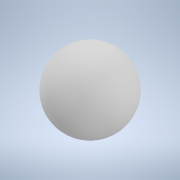
# Autodesk Inventor part: Ball 4mm
Saved by Autodesk Inventor 2021 (Build 250183000, 183)
## iProperties
Created: 2021-08-24
Part Number: Ball 4mm
Material: Genérico
Document SubType Name: Modeling
Designer: Diego.labarca
Density: 1 g/cm^3
Appearance: Valor por defecto
Author: Diego.labarca
Autodesk Inventor part; units mm, degrees
ref_plane "YZ Plane" through (0, 0, 0) normal (1, 0, 0) x (0, 1, 0)
ref_plane "XZ Plane" through (0, 0, 0) normal (0, 1, 0) x (-1, 0, 0)
ref_plane "XY Plane" through (0, 0, 0) normal (0, 0, 1) x (1, 0, 0)
sketch "Boceto1" plane through (0, 0, 0) normal (0, 0, 1) x (1, 0, 0)
  line L0 (0, 2) -> (0, -2)
  line L1 (-0.4, 0) -> (2.4, 0) projected
  arc A0 (0, -2) -> (0, 2) centre (0, 0) ccw
  dimension "d1" = 4
  constraints: 2 end point, 2 point on circle, 1 centre point, 1 coincident, 1 symmetric about line, 1 vertical
  measures "d1" distance of L0.end L0.start
revolve "Revolución1" add sketch "Boceto1" angle 360 about axis through (0, 2, 0) along (0, -1, 0)
